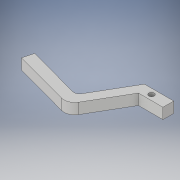
# Autodesk Inventor part: Scissor
Saved by Autodesk Inventor 2019 (Build 230136000, 136)
## iProperties
Created: 2019-01-18
Part Number: Scissor
Material: Generic
Document SubType Name: Modeling
Designer: mar22
Density: 1 g/cm^3
Appearance: Default
Author: mar22
Autodesk Inventor part; units mm, degrees
ref_plane "YZ Plane" through (0, 0, 0) normal (1, 0, 0) x (0, 1, 0)
ref_plane "XZ Plane" through (0, 0, 0) normal (0, 1, 0) x (-1, 0, 0)
ref_plane "XY Plane" through (0, 0, 0) normal (0, 0, 1) x (1, 0, 0)
sketch "Sketch2" plane through (0, 0, 0) normal (0, 1, 0) x (-1, 0, 0)
  line L0 (69.0728, 25.4) -> (127, 25.4)
  line L1 (127, 25.4) -> (179.0216, 114.7196)
  line L2 (207.6006, 126.4556) -> (337.4623, 91.34)
  line L3 (337.4623, 91.34) -> (330.8321, 66.8206)
  line L4 (330.8321, 66.8206) -> (207.3781, 100.2035)
  line L5 (193.0887, 94.3355) -> (138.1457, 0)
  line L6 (138.1457, 0) -> (69.0728, 0)
  arc A0 (207.3781, 100.2035) -> (193.0887, 94.3355) centre (204.063, 87.9438) ccw
  arc A1 (207.6006, 126.4556) -> (179.0216, 114.7196) centre (200.9703, 101.9363) ccw
  line L7 (69.0728, 25.4) -> (69.0728, 0)
  point P0 (0, 0)
  dimension "d6" = 25.4
  dimension "d7" = 12.7
  dimension "d8" = 25.4
  constraints: 16 end point, 4 point on circle, 4 tangent, 2 centre point, 2 parallel, 2 perpendicular
  measures "d6" distance of L2.end L3.end
  measures "d7" radius of A0
  measures "d8" radius of A1
extrude "Extrusion1" add sketch "Sketch2" along normal blind 25.4
sketch "Sketch3" plane through (0, 25.4, 0) normal (0, 1, 0) x (1, 0, 0)
  point P0 (0, 0)
  point P1 (-108.5039, -12.9749)
hole "Hole1" at (-108.5039, 25.4, 12.9749) direction (0, -1, 0) diameter 12.7 depth 38.1 tip angle 118
body "Solid1"
